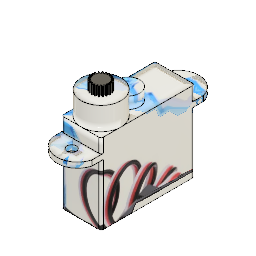
servo motor v1 (Autodesk Fusion 360 design; units mm, degrees)
Autodesk Fusion 360 part; units mm, degrees
note: some values were not read from the file. Set by a fixed rule: which sketch regions a step uses.
sketch "Sketch1" plane through (0, 0, 0) normal (0, 0, 1) x (1, 0, 0)
sketch "Sketch2" plane through (0, 0, 0) normal (0, 0, 1) x (1, 0, 0)
  line L0 (4.25, 10) -> (-4.25, 10)
  line L1 (-4.25, 10) -> (-4.25, -10)
  line L2 (-4.25, -10) -> (4.25, -10)
  line L3 (4.25, -10) -> (4.25, 10)
  line L4 (4.25, 10) -> (-4.25, -10) construction
  line L5 (-4.25, 10) -> (4.25, -10) construction
  dimension "d1" = 8.5
  dimension "d2" = 20
  constraint horizontal L0
  constraint perpendicular L0 L1
  constraint parallel L0 L2
  constraint parallel L1 L3
  constraint coincident L4 origin
  constraint coincident L5 origin
  measures "d1" distance of L1.end L2.end
  measures "d2" distance of L0.end L1.end
extrude "Extrude1" add sketch "Sketch2" along normal blind 13 makes body 1
sketch "Sketch3" plane through (0, 0, 13) normal (0, 0, 1) x (-1, 0, 0)
  line L0 (-4.25, 10) -> (-4.25, -10)
  line L1 (-4.25, -10) -> (4.25, -10)
  line L2 (4.25, -10) -> (4.25, 10)
  line L3 (4.25, 10) -> (-4.25, 10)
  line L4 (-4.25, 11.9334) -> (-4.25, -11.8996)
  line L5 (0, -15.195) -> (0.0324, -15.195)
  line L6 (4.25, -12.0169) -> (4.25, 11.9334)
  line L7 (0, 12.915) -> (0, -12.915)
  arc A0 (4.25, 11.9334) -> (-4.25, 11.9334) centre (0, 10.7952) ccw
  arc A1 (-4.25, -11.8996) -> (4.25, -12.0169) centre (0.0162, -10.7859) ccw
  dimension "d7" = 12.915
  dimension "d8" = 25.83
  constraint parallel L4 L6
  constraint perpendicular L1 L7
  constraint coincident L5.start A1
  constraint coincident A1 L5.end
  measures "d7" distance of origin L7.start
  measures "d8" distance of L7.start L7.end
extrude "Extrude2" add sketch "Sketch3" along normal blind 1.13 bodies 1
sketch "Sketch4" plane through (0, 0, 14.13) normal (0, 0, 1) x (-1, 0, 0)
  arc A0 (-4.25, -11.8996) -> (0, -15.195) centre (0.0162, -10.7859) ccw
  line L0 (0, -15.195) -> (0.0324, -15.195)
  arc A1 (0.0324, -15.195) -> (4.25, -12.0169) centre (0.0162, -10.7859) ccw
  line L1 (4.25, -12.0169) -> (4.25, 11.9334)
  arc A2 (4.25, 11.9334) -> (-4.25, 11.9334) centre (0, 10.7952) ccw
  line L2 (-4.25, 11.9334) -> (-4.25, -11.8996)
  line L3 (4.25, -10) -> (-4.25, -10)
  line L4 (-4.25, -10) -> (-4.25, 10)
  line L5 (-4.25, 10) -> (4.25, 10)
  line L6 (4.25, 10) -> (4.25, -10)
  line L7 (4.25, -10) -> (-4.25, 10) construction
  line L8 (-4.25, -10) -> (4.25, 10) construction
  dimension "d11" = 8.5
  dimension "d12" = 20
  constraint horizontal L3
  constraint perpendicular L3 L4
  constraint parallel L3 L5
  constraint parallel L4 L6
  constraint coincident L7 origin
  constraint coincident L8 origin
  measures "d11" distance of L4.end L5.end
  measures "d12" distance of L3.end L4.end
extrude "Extrude3" add sketch "Sketch4" along normal blind 3 contours L1 L2 L3 L4 L5 L6 bodies 1
sketch "Sketch5" plane through (0, 0, 17.13) normal (0, 0, 1) x (-1, 0, 0)
  line L0 (4.25, 10) -> (-4.25, 10)
  line L1 (-4.25, 10) -> (-4.25, -10)
  line L2 (-4.25, -10) -> (4.25, -10)
  line L3 (4.25, -10) -> (4.25, 10)
  circle A0 centre (0, 5.75) radius 4.25
  constraint tangent L3 A0
  constraint tangent L0 A0
  constraint tangent L1 A0
extrude "Extrude4" add sketch "Sketch5" along normal blind 4.8 contours A0 bodies 1
sketch "Sketch6" plane through (0, 0, 17.13) normal (0, 0, 1) x (-1, 0, 0)
  circle A0 centre (0, 0) radius 2.5
  dimension "d17" = 5
  constraint coincident A0.centre origin
  measures "d17" diameter of A0
extrude "Extrude5" add sketch "Sketch6" along normal blind 2.5 bodies 1
extrude "Extrude6" add 1 faces at (-1.8159, -7.0187, 21.93) along direction (0, 0, 1) blind 0.07 on bodies 1 bodies 1
sketch "Sketch7" plane through (0, 0, 22) normal (0, 0, 1) x (-1, 0, 0)
  circle A0 centre (0, 5.75) radius 4.25
  circle A1 centre (0, 5.75) radius 1.8
  dimension "d22" = 3.6
  constraint concentric A0 A1
  measures "d22" diameter of A1
fillet "Fillet1" radius 0.5 8 edges at (4.25, -10, 6.5) (4.25, 10, 15.63) (4.25, -10, 15.63) (4.25, 10, 6.5) (-4.25, 10, 6.5) (-4.25, 10, 15.63) (-4.25, -10, 15.63) (-4.25, -10, 6.5) on bodies 1
sketch "Sketch1 (2)" plane through (0, 0, 0) normal (0, 0, 1) x (1, 0, 0) in component "Component"
  spline S0 degree 5 poles (2.8944, -0.2439) (2.8944, -0.2439) (2.8944, -0.2439) (2.8945, -0.244) (2.8945, -0.244) (2.8947, -0.244) (2.8948, -0.244) (2.8949, -0.244) (2.8951, -0.244) (2.8953, -0.244) (2.8955, -0.244) (2.8957, -0.244) (2.8959, -0.244) (2.8962, -0.2441) (2.8964, -0.2441) (2.8967, -0.2441) (2.897, -0.2441) (2.8973, -0.2441) (2.8977, -0.2441) (2.898, -0.2441) (2.8984, -0.2441) (2.8987, -0.2441) (2.8991, -0.2442) (2.8995, -0.2442) (2.9, -0.2442) (2.9004, -0.2442) (2.9009, -0.2442) (2.9013, -0.2442) (2.9018, -0.2442) (2.9023, -0.2442) (2.9028, -0.2442) (2.9034, -0.2442) (2.9039, -0.2442) (2.9045, -0.2442) (2.9051, -0.2442) (2.9056, -0.2442) (2.9063, -0.2442) (2.9069, -0.2442) (2.9075, -0.2442) (2.9082, -0.2442) (2.9088, -0.2442) (2.9095, -0.2442) (2.9102, -0.2442) (2.9109, -0.2441) (2.9117, -0.2441) (2.9124, -0.2441) (2.9132, -0.2441) (2.914, -0.2441) (2.9147, -0.244) (2.9156, -0.244) (2.9164, -0.244) (2.9172, -0.2439) (2.9181, -0.2439) (2.9189, -0.2439) (2.9198, -0.2438) (2.9207, -0.2438) (2.9216, -0.2437) (2.9225, -0.2437) (2.9235, -0.2436) (2.9244, -0.2436) (2.9254, -0.2435) (2.9264, -0.2434) (2.9273, -0.2434) (2.9284, -0.2433) (2.9294, -0.2432) (2.9304, -0.2432) (2.9315, -0.2431) (2.9325, -0.243) (2.9336, -0.2429) (2.9347, -0.2428) (2.9358, -0.2427) (2.9369, -0.2426) (2.9381, -0.2425) (2.9392, -0.2424) (2.9404, -0.2423) (2.9415, -0.2422) (2.9427, -0.2421) (2.9439, -0.242) (2.9451, -0.2418) (2.9464, -0.2417) (2.9476, -0.2416) (2.9489, -0.2414) (2.9501, -0.2413) (2.9514, -0.2412) (2.9527, -0.241) (2.954, -0.2409) (2.9554, -0.2407) (2.9567, -0.2405) (2.9581, -0.2404) (2.9594, -0.2402) (2.9608, -0.24) (2.9622, -0.2398) (2.9636, -0.2396) (2.965, -0.2394) (2.9664, -0.2392) (2.9679, -0.239) (2.9693, -0.2388) (2.9708, -0.2386) (2.9723, -0.2384) (2.9738, -0.2382) (2.9753, -0.2379) (2.9768, -0.2377) (2.9783, -0.2375) (2.9799, -0.2372) (2.9814, -0.237) (2.983, -0.2367) (2.9846, -0.2364) (2.9862, -0.2362) (2.9878, -0.2359) (2.9894, -0.2356) (2.991, -0.2353) (2.9927, -0.235) (2.9943, -0.2347) (2.996, -0.2344) (2.9977, -0.2341) (2.9994, -0.2338) (3.0011, -0.2335) (3.0028, -0.2332) (3.0045, -0.2328) (3.0062, -0.2325) (3.008, -0.2321) (3.0098, -0.2318) (3.0115, -0.2314) (3.0133, -0.2311) (3.0151, -0.2307) (3.0169, -0.2303) (3.0188, -0.2299) (3.0206, -0.2295) (3.0224, -0.2291) (3.0243, -0.2287) (3.0262, -0.2283) (3.028, -0.2279) (3.0299, -0.2275) (3.0318, -0.227) (3.0337, -0.2266) (3.0357, -0.2261) (3.0376, -0.2257) (3.0396, -0.2252) (3.0415, -0.2247) (3.0435, -0.2243) (3.0455, -0.2238) (3.0474, -0.2233) (3.0495, -0.2228) (3.0515, -0.2223) (3.0535, -0.2218) (3.0555, -0.2213) (3.0576, -0.2207) (3.0596, -0.2202) (3.0617, -0.2197) (3.0638, -0.2191) (3.0659, -0.2185) (3.068, -0.218) (3.0701, -0.2174) (3.0722, -0.2168) (3.0743, -0.2162) (3.0765, -0.2156) (3.0786, -0.215) (3.0808, -0.2144) (3.0829, -0.2138) (3.0851, -0.2132) (3.0873, -0.2125) (3.0895, -0.2119) (3.0917, -0.2112) (3.0939, -0.2106) (3.0962, -0.2099) (3.0984, -0.2092) (3.1007, -0.2086) (3.1029, -0.2079) (3.1052, -0.2072) (3.1075, -0.2064) (3.1098, -0.2057) (3.1121, -0.205) (3.1144, -0.2043) (3.1167, -0.2035) (3.119, -0.2028) (3.1214, -0.202) (3.1237, -0.2012) (3.1261, -0.2005) (3.1284, -0.1997) (3.1308, -0.1989) (3.1332, -0.1981) (3.1356, -0.1973) (3.138, -0.1964) (3.1404, -0.1956) (3.1428, -0.1948) (3.1453, -0.1939) (3.1477, -0.1931) (3.1502, -0.1922) (3.1526, -0.1913) (3.1551, -0.1904) (3.1576, -0.1895) (3.16, -0.1886) (3.1625, -0.1877) (3.165, -0.1868) (3.1676, -0.1859) (3.1701, -0.1849) (3.1726, -0.184) (3.1751, -0.183) (3.1777, -0.1821) (3.1802, -0.1811) (3.1828, -0.1801) (3.1854, -0.1791) (3.188, -0.1781) (3.1905, -0.1771) (3.1931, -0.1761) (3.1957, -0.175) (3.1983, -0.174) (3.201, -0.1729) (3.2036, -0.1719) (3.2062, -0.1708) (3.2089, -0.1697) (3.2115, -0.1686) (3.2142, -0.1675) (3.2169, -0.1664) (3.2195, -0.1653) (3.2222, -0.1642) (3.2249, -0.163) (3.2276, -0.1619) (3.2303, -0.1607) (3.233, -0.1595) (3.2357, -0.1584) (3.2385, -0.1572) (3.2412, -0.156) (3.244, -0.1548) (3.2467, -0.1536) (3.2495, -0.1523) (3.2522, -0.1511) (3.255, -0.1498) (3.2578, -0.1486) (3.2606, -0.1473) (3.2634, -0.146) (3.2662, -0.1447) (3.269, -0.1434) (3.2718, -0.1421) (3.2746, -0.1408) (3.2774, -0.1395) (3.2803, -0.1381) (3.2831, -0.1368) (3.286, -0.1354) (3.2888, -0.134) (3.2917, -0.1327) (3.294, -0.1315) (3.2957, -0.1307) (3.2969, -0.1301) (3.2974, -0.1298) knots 0 0 0 0 0 0 0.00416667 0.00833333 0.0125 0.01666667 0.02083333 0.025 0.02916667 0.03333333 0.0375 0.04166667 0.04583333 0.05 0.05416667 0.05833333 0.0625 0.06666667 0.07083333 0.075 0.07916667 0.08333333 0.0875 0.09166667 0.09583333 0.1 0.10416667 0.10833333 0.1125 0.11666667 0.12083333 0.125 0.12916667 0.13333333 0.1375 0.14166667 0.14583333 0.15 0.15416667 0.15833333 0.1625 0.16666667 0.17083333 0.175 0.17916667 0.18333333 0.1875 0.19166667 0.19583333 0.2 0.20416667 0.20833333 0.2125 0.21666667 0.22083333 0.225 0.22916667 0.23333333 0.2375 0.24166667 0.24583333 0.25 0.25416667 0.25833333 0.2625 0.26666667 0.27083333 0.275 0.27916667 0.28333333 0.2875 0.29166667 0.29583333 0.3 0.30416667 0.30833333 0.3125 0.31666667 0.32083333 0.325 0.32916667 0.33333333 0.3375 0.34166667 0.34583333 0.35 0.35416667 0.35833333 0.3625 0.36666667 0.37083333 0.375 0.37916667 0.38333333 0.3875 0.39166667 0.39583333 0.4 0.40416667 0.40833333 0.4125 0.41666667 0.42083333 0.425 0.42916667 0.43333333 0.4375 0.44166667 0.44583333 0.45 0.45416667 0.45833333 0.4625 0.46666667 0.47083333 0.475 0.47916667 0.48333333 0.4875 0.49166667 0.49583333 0.5 0.50416667 0.50833333 0.5125 0.51666667 0.52083333 0.525 0.52916667 0.53333333 0.5375 0.54166667 0.54583333 0.55 0.55416667 0.55833333 0.5625 0.56666667 0.57083333 0.575 0.57916667 0.58333333 0.5875 0.59166667 0.59583333 0.6 0.60416667 0.60833333 0.6125 0.61666667 0.62083333 0.625 0.62916667 0.63333333 0.6375 0.64166667 0.64583333 0.65 0.65416667 0.65833333 0.6625 0.66666667 0.67083333 0.675 0.67916667 0.68333333 0.6875 0.69166667 0.69583333 0.7 0.70416667 0.70833333 0.7125 0.71666667 0.72083333 0.725 0.72916667 0.73333333 0.7375 0.74166667 0.74583333 0.75 0.75416667 0.75833333 0.7625 0.76666667 0.77083333 0.775 0.77916667 0.78333333 0.7875 0.79166667 0.79583333 0.8 0.80416667 0.80833333 0.8125 0.81666667 0.82083333 0.825 0.82916667 0.83333333 0.8375 0.84166667 0.84583333 0.85 0.85416667 0.85833333 0.8625 0.86666667 0.87083333 0.875 0.87916667 0.88333333 0.8875 0.89166667 0.89583333 0.9 0.90416667 0.90833333 0.9125 0.91666667 0.92083333 0.925 0.92916667 0.93333333 0.9375 0.94166667 0.94583333 0.95 0.95416667 0.95833333 0.9625 0.96666667 0.97083333 0.975 0.97916667 0.98333333 0.9875 0.99166667 0.99583333 1 1 1 1 1 1
  spline S1 degree 5 poles (2.8944, 0.2439) (2.8944, 0.2439) (2.8944, 0.2439) (2.8945, 0.244) (2.8945, 0.244) (2.8947, 0.244) (2.8948, 0.244) (2.8949, 0.244) (2.8951, 0.244) (2.8953, 0.244) (2.8955, 0.244) (2.8957, 0.244) (2.8959, 0.244) (2.8962, 0.2441) (2.8964, 0.2441) (2.8967, 0.2441) (2.897, 0.2441) (2.8973, 0.2441) (2.8977, 0.2441) (2.898, 0.2441) (2.8984, 0.2441) (2.8987, 0.2441) (2.8991, 0.2442) (2.8995, 0.2442) (2.9, 0.2442) (2.9004, 0.2442) (2.9009, 0.2442) (2.9013, 0.2442) (2.9018, 0.2442) (2.9023, 0.2442) (2.9028, 0.2442) (2.9034, 0.2442) (2.9039, 0.2442) (2.9045, 0.2442) (2.9051, 0.2442) (2.9056, 0.2442) (2.9063, 0.2442) (2.9069, 0.2442) (2.9075, 0.2442) (2.9082, 0.2442) (2.9088, 0.2442) (2.9095, 0.2442) (2.9102, 0.2442) (2.9109, 0.2441) (2.9117, 0.2441) (2.9124, 0.2441) (2.9132, 0.2441) (2.914, 0.2441) (2.9147, 0.244) (2.9156, 0.244) (2.9164, 0.244) (2.9172, 0.2439) (2.9181, 0.2439) (2.9189, 0.2439) (2.9198, 0.2438) (2.9207, 0.2438) (2.9216, 0.2437) (2.9225, 0.2437) (2.9235, 0.2436) (2.9244, 0.2436) (2.9254, 0.2435) (2.9264, 0.2434) (2.9273, 0.2434) (2.9284, 0.2433) (2.9294, 0.2432) (2.9304, 0.2432) (2.9315, 0.2431) (2.9325, 0.243) (2.9336, 0.2429) (2.9347, 0.2428) (2.9358, 0.2427) (2.9369, 0.2426) (2.9381, 0.2425) (2.9392, 0.2424) (2.9404, 0.2423) (2.9415, 0.2422) (2.9427, 0.2421) (2.9439, 0.242) (2.9451, 0.2418) (2.9464, 0.2417) (2.9476, 0.2416) (2.9489, 0.2414) (2.9501, 0.2413) (2.9514, 0.2412) (2.9527, 0.241) (2.954, 0.2409) (2.9554, 0.2407) (2.9567, 0.2405) (2.9581, 0.2404) (2.9594, 0.2402) (2.9608, 0.24) (2.9622, 0.2398) (2.9636, 0.2396) (2.965, 0.2394) (2.9664, 0.2392) (2.9679, 0.239) (2.9693, 0.2388) (2.9708, 0.2386) (2.9723, 0.2384) (2.9738, 0.2382) (2.9753, 0.2379) (2.9768, 0.2377) (2.9783, 0.2375) (2.9799, 0.2372) (2.9814, 0.237) (2.983, 0.2367) (2.9846, 0.2364) (2.9862, 0.2362) (2.9878, 0.2359) (2.9894, 0.2356) (2.991, 0.2353) (2.9927, 0.235) (2.9943, 0.2347) (2.996, 0.2344) (2.9977, 0.2341) (2.9994, 0.2338) (3.0011, 0.2335) (3.0028, 0.2332) (3.0045, 0.2328) (3.0062, 0.2325) (3.008, 0.2321) (3.0098, 0.2318) (3.0115, 0.2314) (3.0133, 0.2311) (3.0151, 0.2307) (3.0169, 0.2303) (3.0188, 0.2299) (3.0206, 0.2295) (3.0224, 0.2291) (3.0243, 0.2287) (3.0262, 0.2283) (3.028, 0.2279) (3.0299, 0.2275) (3.0318, 0.227) (3.0337, 0.2266) (3.0357, 0.2261) (3.0376, 0.2257) (3.0396, 0.2252) (3.0415, 0.2247) (3.0435, 0.2243) (3.0455, 0.2238) (3.0474, 0.2233) (3.0495, 0.2228) (3.0515, 0.2223) (3.0535, 0.2218) (3.0555, 0.2213) (3.0576, 0.2207) (3.0596, 0.2202) (3.0617, 0.2197) (3.0638, 0.2191) (3.0659, 0.2185) (3.068, 0.218) (3.0701, 0.2174) (3.0722, 0.2168) (3.0743, 0.2162) (3.0765, 0.2156) (3.0786, 0.215) (3.0808, 0.2144) (3.0829, 0.2138) (3.0851, 0.2132) (3.0873, 0.2125) (3.0895, 0.2119) (3.0917, 0.2112) (3.0939, 0.2106) (3.0962, 0.2099) (3.0984, 0.2092) (3.1007, 0.2086) (3.1029, 0.2079) (3.1052, 0.2072) (3.1075, 0.2064) (3.1098, 0.2057) (3.1121, 0.205) (3.1144, 0.2043) (3.1167, 0.2035) (3.119, 0.2028) (3.1214, 0.202) (3.1237, 0.2012) (3.1261, 0.2005) (3.1284, 0.1997) (3.1308, 0.1989) (3.1332, 0.1981) (3.1356, 0.1973) (3.138, 0.1964) (3.1404, 0.1956) (3.1428, 0.1948) (3.1453, 0.1939) (3.1477, 0.1931) (3.1502, 0.1922) (3.1526, 0.1913) (3.1551, 0.1904) (3.1576, 0.1895) (3.16, 0.1886) (3.1625, 0.1877) (3.165, 0.1868) (3.1676, 0.1859) (3.1701, 0.1849) (3.1726, 0.184) (3.1751, 0.183) (3.1777, 0.1821) (3.1802, 0.1811) (3.1828, 0.1801) (3.1854, 0.1791) (3.188, 0.1781) (3.1905, 0.1771) (3.1931, 0.1761) (3.1957, 0.175) (3.1983, 0.174) (3.201, 0.1729) (3.2036, 0.1719) (3.2062, 0.1708) (3.2089, 0.1697) (3.2115, 0.1686) (3.2142, 0.1675) (3.2169, 0.1664) (3.2195, 0.1653) (3.2222, 0.1642) (3.2249, 0.163) (3.2276, 0.1619) (3.2303, 0.1607) (3.233, 0.1595) (3.2357, 0.1584) (3.2385, 0.1572) (3.2412, 0.156) (3.244, 0.1548) (3.2467, 0.1536) (3.2495, 0.1523) (3.2522, 0.1511) (3.255, 0.1498) (3.2578, 0.1486) (3.2606, 0.1473) (3.2634, 0.146) (3.2662, 0.1447) (3.269, 0.1434) (3.2718, 0.1421) (3.2746, 0.1408) (3.2774, 0.1395) (3.2803, 0.1381) (3.2831, 0.1368) (3.286, 0.1354) (3.2888, 0.134) (3.2917, 0.1327) (3.294, 0.1315) (3.2957, 0.1307) (3.2969, 0.1301) (3.2974, 0.1298) knots 0 0 0 0 0 0 0.00416667 0.00833333 0.0125 0.01666667 0.02083333 0.025 0.02916667 0.03333333 0.0375 0.04166667 0.04583333 0.05 0.05416667 0.05833333 0.0625 0.06666667 0.07083333 0.075 0.07916667 0.08333333 0.0875 0.09166667 0.09583333 0.1 0.10416667 0.10833333 0.1125 0.11666667 0.12083333 0.125 0.12916667 0.13333333 0.1375 0.14166667 0.14583333 0.15 0.15416667 0.15833333 0.1625 0.16666667 0.17083333 0.175 0.17916667 0.18333333 0.1875 0.19166667 0.19583333 0.2 0.20416667 0.20833333 0.2125 0.21666667 0.22083333 0.225 0.22916667 0.23333333 0.2375 0.24166667 0.24583333 0.25 0.25416667 0.25833333 0.2625 0.26666667 0.27083333 0.275 0.27916667 0.28333333 0.2875 0.29166667 0.29583333 0.3 0.30416667 0.30833333 0.3125 0.31666667 0.32083333 0.325 0.32916667 0.33333333 0.3375 0.34166667 0.34583333 0.35 0.35416667 0.35833333 0.3625 0.36666667 0.37083333 0.375 0.37916667 0.38333333 0.3875 0.39166667 0.39583333 0.4 0.40416667 0.40833333 0.4125 0.41666667 0.42083333 0.425 0.42916667 0.43333333 0.4375 0.44166667 0.44583333 0.45 0.45416667 0.45833333 0.4625 0.46666667 0.47083333 0.475 0.47916667 0.48333333 0.4875 0.49166667 0.49583333 0.5 0.50416667 0.50833333 0.5125 0.51666667 0.52083333 0.525 0.52916667 0.53333333 0.5375 0.54166667 0.54583333 0.55 0.55416667 0.55833333 0.5625 0.56666667 0.57083333 0.575 0.57916667 0.58333333 0.5875 0.59166667 0.59583333 0.6 0.60416667 0.60833333 0.6125 0.61666667 0.62083333 0.625 0.62916667 0.63333333 0.6375 0.64166667 0.64583333 0.65 0.65416667 0.65833333 0.6625 0.66666667 0.67083333 0.675 0.67916667 0.68333333 0.6875 0.69166667 0.69583333 0.7 0.70416667 0.70833333 0.7125 0.71666667 0.72083333 0.725 0.72916667 0.73333333 0.7375 0.74166667 0.74583333 0.75 0.75416667 0.75833333 0.7625 0.76666667 0.77083333 0.775 0.77916667 0.78333333 0.7875 0.79166667 0.79583333 0.8 0.80416667 0.80833333 0.8125 0.81666667 0.82083333 0.825 0.82916667 0.83333333 0.8375 0.84166667 0.84583333 0.85 0.85416667 0.85833333 0.8625 0.86666667 0.87083333 0.875 0.87916667 0.88333333 0.8875 0.89166667 0.89583333 0.9 0.90416667 0.90833333 0.9125 0.91666667 0.92083333 0.925 0.92916667 0.93333333 0.9375 0.94166667 0.94583333 0.95 0.95416667 0.95833333 0.9625 0.96666667 0.97083333 0.975 0.97916667 0.98333333 0.9875 0.99166667 0.99583333 1 1 1 1 1 1
  spline S2 degree 5 poles (2.8942, -0.2439) (2.8942, -0.2439) (2.8942, -0.2439) (2.8942, -0.2439) (2.8943, -0.2439) (2.8943, -0.2439) (2.8943, -0.2439) (2.8943, -0.2439) (2.8943, -0.2439) (2.8944, -0.2439) knots 0 0 0 0 0 0 0.2 0.4 0.6 0.8 1 1 1 1 1 1
  spline S3 degree 5 poles (2.8942, 0.2439) (2.8942, 0.2439) (2.8942, 0.2439) (2.8942, 0.2439) (2.8943, 0.2439) (2.8943, 0.2439) (2.8943, 0.2439) (2.8943, 0.2439) (2.8943, 0.2439) (2.8944, 0.2439) knots 0 0 0 0 0 0 0.2 0.4 0.6 0.8 1 1 1 1 1 1
  line L0 (0, 0) -> (2.8942, -0.2439)
  line L1 (0, 0) -> (2.8942, 0.2439)
  arc A0 (3.2974, -0.1298) -> (3.2974, 0.1298) centre (0, 0) ccw
  point P0 (2.8949, -0.244)
  point P1 (2.8958, -0.244)
  point P2 (2.897, -0.2441)
  point P3 (2.8986, -0.2441)
  point P4 (2.9005, -0.2442)
  point P5 (2.9028, -0.2442)
  point P6 (2.9054, -0.2442)
  point P7 (2.9084, -0.2442)
  point P8 (2.9118, -0.2441)
  point P9 (2.9155, -0.244)
  point P10 (2.9195, -0.2438)
  point P11 (2.9239, -0.2436)
  point P12 (2.9286, -0.2433)
  point P13 (2.9337, -0.2429)
  point P14 (2.9392, -0.2424)
  point P15 (2.9449, -0.2419)
  point P16 (2.9511, -0.2412)
  point P17 (2.9575, -0.2404)
  point P18 (2.9643, -0.2395)
  point P19 (2.9715, -0.2385)
  point P20 (2.979, -0.2374)
  point P21 (2.9868, -0.2361)
  point P22 (2.9949, -0.2346)
  point P23 (3.0034, -0.233)
  point P24 (3.0122, -0.2313)
  point P25 (3.0213, -0.2294)
  point P26 (3.0308, -0.2273)
  point P27 (3.0405, -0.225)
  point P28 (3.0506, -0.2225)
  point P29 (3.061, -0.2198)
  point P30 (3.0717, -0.217)
  point P31 (3.0827, -0.2139)
  point P32 (3.094, -0.2106)
  point P33 (3.1057, -0.207)
  point P34 (3.1176, -0.2032)
  point P35 (3.1298, -0.1992)
  point P36 (3.1423, -0.195)
  point P37 (3.155, -0.1905)
  point P38 (3.1681, -0.1857)
  point P39 (3.1814, -0.1806)
  point P40 (3.195, -0.1753)
  point P41 (3.2089, -0.1697)
  point P42 (3.223, -0.1638)
  point P43 (3.2374, -0.1576)
  point P44 (3.2521, -0.1512)
  point P45 (3.2669, -0.1444)
  point P46 (3.2821, -0.1373)
  point P47 (2.8949, 0.244)
  point P48 (2.8958, 0.244)
  point P49 (2.897, 0.2441)
  point P50 (2.8986, 0.2441)
  point P51 (2.9005, 0.2442)
  point P52 (2.9028, 0.2442)
  point P53 (2.9054, 0.2442)
  point P54 (2.9084, 0.2442)
  point P55 (2.9118, 0.2441)
  point P56 (2.9155, 0.244)
  point P57 (2.9195, 0.2438)
  point P58 (2.9239, 0.2436)
  point P59 (2.9286, 0.2433)
  point P60 (2.9337, 0.2429)
  point P61 (2.9392, 0.2424)
  point P62 (2.9449, 0.2419)
  point P63 (2.9511, 0.2412)
  point P64 (2.9575, 0.2404)
  point P65 (2.9643, 0.2395)
  point P66 (2.9715, 0.2385)
  point P67 (2.979, 0.2374)
  point P68 (2.9868, 0.2361)
  point P69 (2.9949, 0.2346)
  point P70 (3.0034, 0.233)
  point P71 (3.0122, 0.2313)
  point P72 (3.0213, 0.2294)
  point P73 (3.0308, 0.2273)
  point P74 (3.0405, 0.225)
  point P75 (3.0506, 0.2225)
  point P76 (3.061, 0.2198)
  point P77 (3.0717, 0.217)
  point P78 (3.0827, 0.2139)
  point P79 (3.094, 0.2106)
  point P80 (3.1057, 0.207)
  point P81 (3.1176, 0.2032)
  point P82 (3.1298, 0.1992)
  point P83 (3.1423, 0.195)
  point P84 (3.155, 0.1905)
  point P85 (3.1681, 0.1857)
  point P86 (3.1814, 0.1806)
  point P87 (3.195, 0.1753)
  point P88 (3.2089, 0.1697)
  point P89 (3.223, 0.1638)
  point P90 (3.2374, 0.1576)
  point P91 (3.2521, 0.1512)
  point P92 (3.2669, 0.1444)
  point P93 (3.2821, 0.1373)
sketch "Sketch2 (2)" plane through (0, 0, 0) normal (0, 0, 1) x (1, 0, 0) in component "Component"
  circle A0 centre (0, 0) radius 2.625
extrude "Extrude1'" add sketch "Sketch2 (2)" along normal blind 2 separate body makes body 2 in component "Component"
extrude "Extrude2'" add sketch "Sketch1 (2)" along normal blind 2 separate body makes body 3 in component "Component"
pattern_circular "C-Pattern1" count 20 over 360 about axis through (0, 0, 1.75) along (0, 0, 1) of "Extrude2'" makes body 4 makes body 5 makes body 6 makes body 7 makes body 8 makes body 9 makes body 10 makes body 11 makes body 12 makes body 13 makes body 14 makes body 15 makes body 16 makes body 17 makes body 18 makes body 19 makes body 20 makes body 21 makes body 22 in component "Component"
combine "Combine1" operation add target body 2 tool bodies 3 4 5 6 7 8 9 10 11 12 13 14 15 16 17 18 19 20 21 22 in component "Component"
sketch "Sketch3 (2)" plane through (0, 0, 0) normal (0, 0, 1) x (1, 0, 0) in component "Component"
  line L0 (0, 0) -> (48.2432, 0) construction
  line L1 (48.2432, 0) -> (48.2432, 3) construction
  line L2 (48.2432, 3) -> (0, 3) construction
  line L3 (0, 3) -> (0, 0) construction
  constraint perpendicular L0 L1
  constraint parallel L0 L2
  constraint parallel L1 L3
move_body "Move1" bodies 2 to x (1, 0, 0) y (0, 1, 0) z (0, 0, 1) at (0, 0, 40) in component "Component"
move_body "Move2" bodies 2 to x (1, 0, 0) y (0, 1, 0) z (0, 0, 1) at (-0.0245, -5.8288, -18) in component "Component"
scale "Scale1" factor 0.6 about (2.1736, -3.9303, 24) bodies 2 in component "Component"
move_body "Move3" bodies 2 to x (1, 0, 0) y (0, 1, 0) z (0, 0, 1) at (-0.8718, -0.7323, -0.5) in component "Component"
extrude "Extrude3'" add 1 faces at (-0.4211, -6.0943, 23.5) along direction (0, 0, 1) blind 0.9 on bodies 2 bodies 2 in component "Component"
move_body "Move4" bodies 2 to x (1, 0, 0) y (0, 1, 0) z (0, 0, 1) at (0, 0, -0.5) in component "Component"
sketch "Sketch8" plane through (0, 0, 14.13) normal (0, 0, 1) x (-1, 0, 0)
  line L0 (-3.75, 10) -> (3.75, 10)
  arc A0 (4.25, 9.5) -> (3.75, 10) centre (3.75, 9.5) ccw
  line L1 (4.25, 9.5) -> (4.25, 11.9334)
  arc A1 (4.25, 11.9334) -> (-4.25, 11.9334) centre (0, 10.7952) ccw
  line L2 (-4.25, 11.9334) -> (-4.25, 9.5)
  arc A2 (-3.75, 10) -> (-4.25, 9.5) centre (-3.75, 9.5) ccw
  circle A3 centre (0.0191, 12.0131) radius 1
  dimension "d34" = 2
  measures "d34" diameter of A3
sketch "Sketch9" plane through (0, 0, 14.13) normal (0, 0, 1) x (-1, 0, 0)
  line L0 (3.75, -10) -> (-3.75, -10)
  arc A0 (-4.25, -9.5) -> (-3.75, -10) centre (-3.75, -9.5) ccw
  line L1 (-4.25, -9.5) -> (-4.25, -11.8996)
  arc A1 (-4.25, -11.8996) -> (0, -15.195) centre (0.0162, -10.7859) ccw
  line L2 (0, -15.195) -> (0.0324, -15.195)
  arc A2 (0.0324, -15.195) -> (4.25, -12.0169) centre (0.0162, -10.7859) ccw
  line L3 (4.25, -12.0169) -> (4.25, -9.5)
  arc A3 (3.75, -10) -> (4.25, -9.5) centre (3.75, -9.5) ccw
  circle A4 centre (0.1077, -12.0031) radius 1
  dimension "d35" = 2
  measures "d35" diameter of A4
extrude "Extrude7" cut sketch "Sketch9" sketch "Sketch8" against normal blind 6 contours A4 of sketch 2 contours A3 bodies 1
copy_body "Body->Comp1" bodies 1 removing the originals makes body 23 in component "Component'"
component "Component" placed x (1, 0, 0) y (0, 1, 0) z (0, 0, 1) at (0, 0, 0)
component "Component'" placed x (1, 0, 0) y (0, 1, 0) z (0, 0, 1) at (0, 0, 0)
component "3.7g servo" placed x (1, 0, 0) y (0, 1, 0) z (0, 0, 1) at (0, 0, 0)
